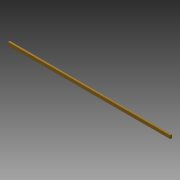
# Autodesk Inventor part: relsa2
Saved by Autodesk Inventor 2015 (Build 190159000, 159)
## iProperties
Created: 2016-04-26
Part Number: relsa2
Material: Brass, Soft Yellow
Document SubType Name: Modeling
Designer: Kostya
Density: 8.47 g/cm^3
Appearance: Brass - Satin
Author: Kostya
Autodesk Inventor part; units mm, degrees
ref_plane "YZ Plane" through (0, 0, 0) normal (1, 0, 0) x (0, 1, 0)
ref_plane "XZ Plane" through (0, 0, 0) normal (0, 1, 0) x (-1, 0, 0)
ref_plane "XY Plane" through (0, 0, 0) normal (0, 0, 1) x (1, 0, 0)
sketch "Sketch1" plane through (0, 0, 0) normal (0, 1, 0) x (-1, 0, 0)
  line L0 (0, 0) -> (0, -10)
  line L1 (0, -10) -> (500, -10)
  line L2 (500, -10) -> (500, 0)
  line L3 (500, 0) -> (0, 0)
  dimension "d0" = 10
  dimension "d1" = 500
  dimension "d2" = 500
  constraints: 8 end point, 2 perpendicular, 2 vertical
  measures "d0" distance of L0.start L0.end
  measures "d1" distance of L0.end L1.end
  measures "d2" distance of L2.end L0.start
extrude "Extrusion1" add sketch "Sketch1" along normal blind 5
sketch "Sketch2" plane through (0, 0, 0) normal (0, -1, 0) x (1, 0, 0)
  point P0 (-485, -5)
hole "Hole1" at (-485, 0, -5) direction (0, 1, 0) diameter 5.5 depth 5 countersink diameter 10.4 countersink angle 90
sketch "Sketch3" plane through (0, 0, 0) normal (0, -1, 0) x (1, 0, 0)
  point P0 (-15, -5)
hole "Hole3" at (-15, 0, -5) direction (0, 1, 0) diameter 5.5 depth 5 countersink diameter 10.4 countersink angle 90
body "Solid1"
